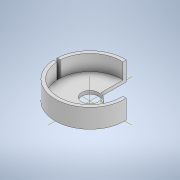
# Autodesk Inventor part: base layer 3
Saved by Autodesk Inventor 2022 (Build 260153000, 153)
## iProperties
Created: 2021-07-05
Part Number: base layer 3
Material: Generic
Document SubType Name: Modeling
Designer: Alicia
Density: 1 g/cm^3
Appearance: Default
Mass: 1.77348 g
Surface Area: 35.637 cm^2
Volume: 1.77348 cm^3
Author: Alicia
Autodesk Inventor part; units mm, degrees
ref_plane "YZ Plane" through (0, 0, 0) normal (1, 0, 0) x (0, 1, 0)
ref_plane "XZ Plane" through (0, 0, 0) normal (0, 1, 0) x (-1, 0, 0)
ref_plane "XY Plane" through (0, 0, 0) normal (0, 0, 1) x (1, 0, 0)
sketch "Sketch9" plane through (0, 0, 0) normal (0, 1, 0) x (-1, 0, 0)
  line L0 (21, 0) -> (-21, 0) construction
  line L1 (0, 21) -> (0, -21) construction
  line L2 (21, -1) -> (20.9762, -1)
  line L3 (21, 1) -> (20.9762, 1)
  line L4 (-20.9762, 1) -> (-21, 1)
  line L5 (1, 21) -> (1, 20.9762)
  line L6 (1, -20.9762) -> (1, -21)
  line L7 (-1, 21) -> (-1, 20.9762)
  line L8 (-1, -5.9161) -> (-1, -21)
  line L9 (-5.9161, -1) -> (-18.9762, -1)
  circle A0 centre (0, 0) radius 5
  arc A1 (-5.9161, -1) -> (-1, -5.9161) centre (0, 0) ccw
  line L10 (-20.9762, -1) -> (-18.9762, -1)
  line L11 (1, -21) -> (1, -3.873) construction
  line L12 (-3.873, 1) -> (-18.9762, 1) construction
  line L13 (-18.9762, 1) -> (-20.9762, 1) construction
  line L14 (-3.873, 1) -> (20.9762, 1) construction
  line L15 (-5.9161, -1) -> (20.9762, -1) construction
  line L16 (1, -3.873) -> (1, 20.9762) construction
  line L17 (-1, -5.9161) -> (-1, 20.9762) construction
  line L18 (0, 21) -> (0, 19) construction
  line L19 (0, 19) -> (1, 19) construction
  arc A2 (-1, -20.9762) -> (0, 21) centre (0, 0) ccw construction
  arc A3 (20.9762, 1) -> (-20.9762, -1) centre (0, 0) ccw construction
  arc A4 (-1, -18.9737) -> (-18.9737, -1) centre (0, 0) ccw
  line L20 (-1, 19) -> (1, 19)
  point P0 (-4.899, -1)
  point P1 (-1, -4.899)
  dimension "d35" = 10
  dimension "d50" = 2
  dimension "d53" = 38
  constraints: 42 end point, 22 point on circle, 10 parallel, 8 point on line, 5 centre point, 4 coincident, 3 perpendicular, 1 collinear, 1 horizontal, 1 other
  measures "d35" diameter of A0
  measures "d50" distance between parallel lines of L9 L12
  measures "d53" diameter of A4
extrude "Extrusion5" add sketch "Sketch9" along normal blind 2
chamfer "Chamfer1" distance 0.5 distance2 1 1 edges at (4.2426, 2, -4.2426) measured on face at (13.5988, 2, 4.219)
sketch "Sketch12" plane through (0, 0, 0) normal (0, 1, 0) x (-1, 0, 0)
  circle A0 centre (0, 0) radius 5 projected
  arc A1 (-1, -18.9737) -> (-18.9737, -1) centre (0, 0) ccw
  line L0 (-18.9737, -1) -> (-5.4083, -1) projected
  line L1 (-18.9737, -1) -> (-20.9762, -1)
  line L2 (-1, -5.4083) -> (-1, -18.9737) projected
  line L3 (-1, -18.9737) -> (-1, -20.9762)
  line L4 (-20.9762, -1) -> (20.9762, -1) construction
  line L5 (-20.9762, 1) -> (20.9762, 1) construction
  line L6 (20.9762, 1) -> (18.9762, 1)
  line L7 (20.9762, -1) -> (18.9762, -1)
  line L8 (18.9762, -1) -> (18.9762, 1)
  arc A2 (-1, -20.9762) -> (20.9762, -1) centre (0, 0) ccw
  arc A3 (20.9762, 1) -> (-20.9762, -1) centre (0, 0) ccw
  point P0 (18.9762, 0.9512)
  point P1 (18.9762, -0.9512)
  dimension "d60" = 19
  dimension "d63" = 2
  dimension "d64" = 2
  dimension "d65" = 2
  constraints: 14 end point, 6 point on circle, 3 centre point, 3 point on line, 2 coincident, 2 collinear, 1 parallel, 1 perpendicular
  measures "d60" radius of A1
  measures "d63" distance between parallel lines of L4 L5
  measures "d64" distance of L5.end L6.end
  measures "d65" distance of L4.end L7.end
extrude "Extrusion8" add sketch "Sketch12" along normal blind 11.5 contours A1 L1 A3 L6 L8 | A1 L8 L7 A2 L3
body "Solid2"
